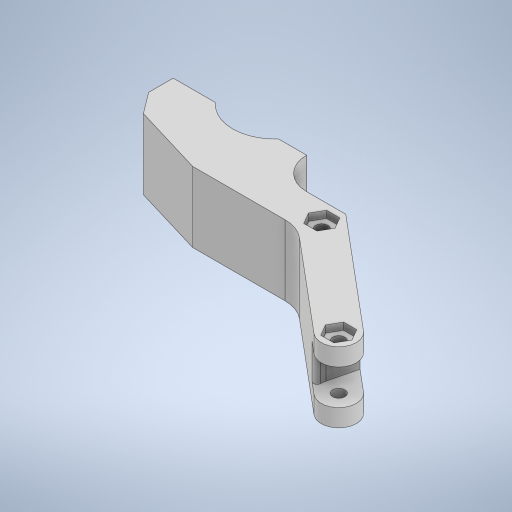
# Autodesk Inventor part: Claw_R
Saved by Autodesk Inventor 2023 (Build 270158000, 158)
## iProperties
Created: 2024-07-18
Part Number: Claw_R
Material: Generic
Document SubType Name: Modeling
Designer: Swoby
Density: 1 g/cm^3
Appearance: Default
Author: Swoby
Autodesk Inventor part; units mm, degrees
ref_plane "YZ Plane" through (0, 0, 0) normal (1, 0, 0) x (0, 1, 0)
ref_plane "XZ Plane" through (0, 0, 0) normal (0, 1, 0) x (-1, 0, 0)
ref_plane "XY Plane" through (0, 0, 0) normal (0, 0, 1) x (1, 0, 0)
sketch "Sketch1" plane through (0, 0, 0) normal (0, 1, 0) x (-1, 0, 0)
  arc A0 (10, -14) -> (1, -5) centre (1, -14) ccw
  line L0 (10, -14) -> (18, -14)
  arc A1 (36, -14) -> (18, -14) centre (27, -21.9373) ccw
  line L1 (36, -14) -> (48, -14)
  line L2 (23.5, 5) -> (43.5, -1)
  line L3 (43.5, -1) -> (48, -7)
  line L4 (48, -7) -> (48, -14)
  circle A2 centre (-8.3199, 0) radius 1.75
  circle A3 centre (-38.3199, 25.173) radius 1.75
  line L5 (-38.3199, 25.173) -> (-8.3199, 0) construction
  line L6 (-8.3199, 0) -> (0, 0) construction
  line L7 (-41.5338, 21.3428) -> (-10.1397, -5)
  arc A4 (-35.1059, 29.0032) -> (-41.5338, 21.3428) centre (-38.3199, 25.173) ccw
  line L8 (1, -5) -> (-10.1397, -5)
  line L9 (-35.1059, 29.0032) -> (-6.5, 5)
  line L10 (-6.5, 5) -> (23.5, 5)
  point P0 (-25.8367, 8.1714)
  point P1 (-23.3199, 12.5865)
  dimension "d3" = 1
  dimension "d8" = 12
  dimension "d9" = 8
  dimension "d10" = 18
  dimension "d11" = 9
  dimension "d12" = 9
  dimension "d13" = 12
  dimension "d24" = 3.5
  dimension "d25" = 3.5
  dimension "d26" = 140
  dimension "d36" = 5
  dimension "d38" = 9
  dimension "d40" = 5
  dimension "d41" = 30
  dimension "d54" = 5
  dimension "d55" = 5
  dimension "d56" = 7
  dimension "d57" = 30
  dimension "d58" = 20
  dimension "d59" = 4.5
  dimension "d60" = 6
  dimension "d61" = 6
  constraints: 22 end point, 6 point on circle, 5 centre point, 3 horizontal, 3 parallel, 2 midpoint, 1 coincident, 1 collinear, 1 vertical
  measures "d3" horizontal distance of L6.end L8.start
  measures "d8" distance of L1.start L1.end
  measures "d9" distance of L0.start L0.end
  measures "d10" distance of L0.end L1.start
  measures "d11" horizontal distance of L8.start L0.start
  measures "d12" horizontal distance of L8.start L0.start
  measures "d13" radius of A1
  measures "d24" diameter of A2
  measures "d25" diameter of A3
  measures "d26" angle of L5 L6
  measures "d36" distance between parallel lines of L8 L6
  measures "d38" radius of A0
  measures "d40" radius of A4
  measures "d41" horizontal distance of L5.start L5.end
  measures "d54" distance between parallel lines of L5 L9
  measures "d55" distance between parallel lines of L7 L5
  measures "d56" distance of L3.end L1.end
  measures "d57" distance of L9.end L2.start
  measures "d58" horizontal distance of L2.start L2.end
  measures "d59" horizontal distance of L2.end L3.end
  measures "d60" vertical distance of L3.end L2.end
  measures "d61" vertical distance of L2.end L2.start
extrude "Extrusion1" add sketch "Sketch1" along normal blind 20 contours A0 L8 L7 A4 L9 L10 L2 L3 L4 L1 A1 L0 | A2 | A3
sketch "Sketch2" plane through (10.1397, 0, -5) normal (0, 0, -1) x (-1, 0, 0)
  line L0 (-33.1801, 0) -> (-33.1801, 20) projected
  line L1 (-33.1801, 15) -> (6.8199, 15)
  line L2 (6.8199, 15) -> (6.8199, 5)
  line L3 (6.8199, 5) -> (-33.1801, 5)
  line L4 (-33.1801, 5) -> (-33.1801, 15)
  line L5 (-31.3941, 20) -> (0, 20) projected
  line L6 (-31.3941, 0) -> (0, 0) projected
  point P0 (10.1397, 0)
  dimension "d47" = 5
  dimension "d48" = 5
  dimension "d49" = 40
  constraints: 8 end point, 2 parallel, 1 horizontal, 1 perpendicular, 1 point on line
  measures "d47" distance between parallel lines of L1 L5
  measures "d48" distance between parallel lines of L6 L3
  measures "d49" distance of L1.start L1.end
extrude "Extrusion2" cut sketch "Sketch2" against normal through all
extrude "Extrusion3" cut sketch "Sketch1" along normal through all contours A2 | A3
fillet "Fillet1" radius 10 2 edges at (6.5, 17.5, 5) (6.5, 2.5, 5)
sketch "Sketch3" plane through (0, 0, 0) normal (0, -1, 0) x (1, 0, 0)
  circle A0 centre (38.3199, 25.173) radius 1.75 construction
  circle A1 centre (8.3199, 0) radius 1.75 construction
  line L0 (-48, -14) -> (-48, -7) construction
  line L1 (-36, -14) -> (-48, -14) construction
  arc A2 (-18, -14) -> (-36, -14) centre (-27, -21.9373) ccw construction
  line L2 (-10, -14) -> (-18, -14) construction
  arc A3 (-1, -5) -> (-10, -14) centre (-1, -14) ccw construction
  line L3 (10.1397, -5) -> (-1, -5) construction
  line L4 (41.5338, 21.3428) -> (10.1397, -5) construction
  arc A4 (41.5338, 21.3428) -> (35.1059, 29.0032) centre (38.3199, 25.173) ccw construction
  line L5 (9.2748, 7.3284) -> (35.1059, 29.0032) construction
  arc A5 (3.3199, 5) -> (9.2748, 7.3284) centre (2.847, 14.9888) ccw construction
  line L6 (-23.5, 5) -> (2.8603, 5) construction
  line L7 (-43.5, -1) -> (-23.5, 5) construction
  line L8 (-48, -7) -> (-43.5, -1) construction
  circle A6 centre (8.3199, 0) radius 3.25
  circle A7 centre (38.3199, 25.173) radius 3.25
  line L9 (3.3199, 5.0106) -> (3.3199, 5) projected
  arc A8 (2.8603, 5) -> (3.3199, 5.0106) centre (2.8603, 15) ccw projected
  point P0 (0, 0)
  dimension "d63" = 6.5
  dimension "d64" = 6.5
  constraints: 2 centre point, 2 coincident
  measures "d63" diameter of A6
  measures "d64" diameter of A7
extrude "Extrusion4" cut sketch "Sketch3" against normal blind 2
sketch "Sketch4" plane through (0, 20, 0) normal (0, 1, 0) x (1, 0, 0)
  circle A0 centre (8.3199, 0) radius 1.75 projected
  circle A1 centre (38.3199, -25.173) radius 1.75 projected
  line L0 (6.4435, 3.25) -> (10.1962, 3.25)
  line L1 (10.1962, 3.25) -> (12.0726, 0)
  line L2 (12.0726, 0) -> (10.1962, -3.25)
  line L3 (10.1962, -3.25) -> (6.4435, -3.25)
  line L4 (6.4435, -3.25) -> (4.5671, 0)
  line L5 (4.5671, 0) -> (6.4435, 3.25)
  line L6 (36.4435, -21.923) -> (40.1962, -21.923)
  line L7 (40.1962, -21.923) -> (42.0726, -25.173)
  line L8 (42.0726, -25.173) -> (40.1962, -28.423)
  line L9 (40.1962, -28.423) -> (36.4435, -28.423)
  line L10 (36.4435, -28.423) -> (34.5671, -25.173)
  line L11 (34.5671, -25.173) -> (36.4435, -21.923)
  point P0 (0, 0)
  point P1 (8.3199, 3.25)
  point P2 (8.3199, -3.25)
  dimension "d67" = 6.5
  dimension "d68" = 6.5
  constraints: 24 end point, 2 coincident, 2 horizontal, 2 midpoint, 26 other
  measures "d67" distance between parallel lines of L6 L9
  measures "d68" distance of point (8.32, 3.25) point (8.32, -3.25)
extrude "Extrusion5" cut sketch "Sketch4" against normal blind 2 contours A0 | L0 L1 L2 L3 L4 L5 | L6 L7 L8 L9 L10 L11
sketch "Sketch5" plane through (0, 0, 0) normal (0, -1, 0) x (1, 0, 0)
  circle A0 centre (38.3199, 25.173) radius 3.25 projected
  circle A1 centre (8.3199, 0) radius 3.25 projected
  line L0 (-48, -14) -> (-48, -7) projected
  line L1 (-36, -14) -> (-48, -14) projected
  arc A2 (-18, -14) -> (-36, -14) centre (-27, -21.9373) ccw projected
  line L2 (-10, -14) -> (-18, -14) projected
  arc A3 (-1, -5) -> (-10, -14) centre (-1, -14) ccw projected
  line L3 (10.1397, -5) -> (-1, -5) projected
  line L4 (41.5338, 21.3428) -> (10.1397, -5) projected
  arc A4 (41.5338, 21.3428) -> (35.1059, 29.0032) centre (38.3199, 25.173) ccw projected
  line L5 (9.2748, 7.3284) -> (35.1059, 29.0032) projected
  arc A5 (3.3199, 5) -> (9.2748, 7.3284) centre (2.847, 14.9888) ccw projected
  line L6 (-23.5, 5) -> (2.8603, 5) projected
  line L7 (-43.5, -1) -> (-23.5, 5) projected
  line L8 (-48, -7) -> (-43.5, -1) projected
  line L9 (17.6621, 1.3121) -> (11.2343, 8.9725)
  line L10 (11.2343, 8.9725) -> (28.9776, 23.8609)
  line L11 (28.9776, 23.8609) -> (35.4054, 16.2005)
  line L12 (35.4054, 16.2005) -> (17.6621, 1.3121)
  line L13 (3.3199, 5.0106) -> (3.3199, 5) projected
  arc A6 (2.8603, 5) -> (3.3199, 5.0106) centre (2.8603, 15) ccw projected
  point P0 (0, 0)
  dimension "d71" = 8
  dimension "d72" = 8
  constraints: 8 end point, 4 point on line, 2 perpendicular, 1 collinear
  measures "d71" distance from line of L9 A1.centre
  measures "d72" distance from line of A0.centre L11
extrude "Extrusion6" add sketch "Sketch5" against normal up to surface (20 mm away) contours L9 L5 L11 L4
chamfer "Chamfer1" distance 3 angle 45 1 edges at (17.6621, 10, 1.3121)
sketch "Sketch6" plane through (3.3199, 15, -5) normal (0, -1, 0) x (1, 0, 0)
  line L0 (12.4139, 8.6102) -> (7.9144, 13.9725) projected
  line L1 (5.9683, 12.3396) -> (7.9144, 13.9725) projected
  arc A0 (0, 10.0106) -> (5.9683, 12.3396) centre (-0.4596, 20) ccw projected
  line L2 (6.8199, 0) -> (0, 0) projected
  line L3 (16.6404, 8.2404) -> (6.8199, 0) projected
  line L4 (12.4139, 8.6102) -> (16.6404, 8.2404) projected
  circle A1 centre (5, 5) radius 1.75 projected
  line L5 (12.4139, 8.6102) -> (2.1743, 9.5061)
  arc A2 (2.1743, 9.5061) -> (0, 7.5137) centre (2, 7.5137) ccw
  line L6 (0, 0) -> (0, 10.0106) projected
  point P0 (-3.3199, 5)
  point P1 (0, 7.5137)
  dimension "d78" = 2
  constraints: 2 end point, 2 point on circle, 1 centre point, 1 collinear, 1 tangent
  measures "d78" radius of A2
extrude "Extrusion7" add sketch "Sketch6" along normal up to surface (15 mm away) contours L5 A2 L6 A0 L1 L0
sketch "Sketch7" plane through (38.3199, 15, 25.173) normal (0, -1, 0) x (0.7660444, 0, 0.6427876)
  line L0 (-8, 5) -> (-8, -5) projected
  line L1 (0, -5) -> (-8, -5) projected
  arc A0 (0, -5) -> (0, 5) centre (0, 0) ccw projected
  line L2 (-8, 5) -> (0, 5) projected
  circle A1 centre (0, 0) radius 1.75 projected
  circle A2 centre (0, 0) radius 5
  line L3 (-8, -5) -> (-4.4944, 2.191)
  point P0 (-45.5356, 5.3479)
  point P1 (0, 5)
  constraints: 2 coincident, 2 end point, 5 other
extrude "Extrusion8" add sketch "Sketch7" along normal up to surface (10 mm away) contours L2 A2 L3 L0
fillet "Fillet2" radius 1 1 edges at (35.1059, 10, 29.0032)
equation "\"d63\" = d64"
equation "\"d68\" = d67"
body "Solid1"
